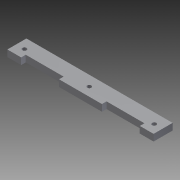
# Autodesk Inventor part: carro x lado motor pieza 3
Saved by Autodesk Inventor 2012 (Build 160160000, 160)
## iProperties
Created: 2014-12-17
Part Number: carro x lado motor pieza 3
Material: Default
Document SubType Name: Modeling
Designer: PRINCIPAL
Density: 1 g/cm^3
Author: PRINCIPAL
Autodesk Inventor part; units mm, degrees
ref_plane "YZ Plane" through (0, 0, 0) normal (1, 0, 0) x (0, 1, 0)
ref_plane "XZ Plane" through (0, 0, 0) normal (0, 1, 0) x (-1, 0, 0)
ref_plane "XY Plane" through (0, 0, 0) normal (0, 0, 1) x (1, 0, 0)
sketch "Boceto1" plane through (0, 0, 0) normal (0, 0, 1) x (1, 0, 0)
  arc A0 (-67.1173, 21.3488) -> (-68.6673, 19.7988) centre (-67.1173, 19.7988) ccw
  arc A1 (-68.6673, 19.7988) -> (-67.1173, 18.2488) centre (-67.1173, 19.7988) ccw
  arc A2 (-67.1173, 18.2488) -> (-65.5673, 19.7988) centre (-67.1173, 19.7988) ccw
  arc A3 (-65.5673, 19.7988) -> (-67.1173, 21.3488) centre (-67.1173, 19.7988) ccw
  arc A4 (-116.1173, 21.3488) -> (-117.6673, 19.7988) centre (-116.1173, 19.7988) ccw
  arc A5 (-117.6673, 19.7988) -> (-116.1173, 18.2488) centre (-116.1173, 19.7988) ccw
  arc A6 (-116.1173, 18.2488) -> (-114.5673, 19.7988) centre (-116.1173, 19.7988) ccw
  arc A7 (-114.5673, 19.7988) -> (-116.1173, 21.3488) centre (-116.1173, 19.7988) ccw
  arc A8 (-18.1173, 21.3488) -> (-19.6673, 19.7988) centre (-18.1173, 19.7988) ccw
  arc A9 (-19.6673, 19.7988) -> (-18.1173, 18.2488) centre (-18.1173, 19.7988) ccw
  arc A10 (-18.1173, 18.2488) -> (-16.5673, 19.7988) centre (-18.1173, 19.7988) ccw
  arc A11 (-16.5673, 19.7988) -> (-18.1173, 21.3488) centre (-18.1173, 19.7988) ccw
  line L0 (-50.9173, 13.119) -> (-50.9173, 16.5988)
  line L1 (-50.9173, 16.5988) -> (-22.3173, 16.5988)
  line L2 (-22.3173, 16.5988) -> (-22.3173, 13.119)
  line L3 (-22.3173, 13.119) -> (-11.9173, 13.119)
  line L4 (-11.9173, 13.119) -> (-11.9173, 27.4988)
  line L5 (-11.9173, 27.4988) -> (-122.3173, 27.4988)
  line L6 (-122.3173, 27.4988) -> (-122.3173, 13.119)
  line L7 (-122.3173, 13.119) -> (-111.9173, 13.119)
  line L8 (-111.9173, 13.119) -> (-111.9173, 16.5988)
  line L9 (-111.9173, 16.5988) -> (-83.3173, 16.5988)
  line L10 (-83.3173, 16.5988) -> (-83.3173, 13.119)
  line L11 (-83.3173, 13.119) -> (-50.9173, 13.119)
  point P0 (0, 0)
  constraints: 24 end point, 24 point on circle, 12 centre point
extrude "Extrusión1" add sketch "Boceto1" along normal blind 5
